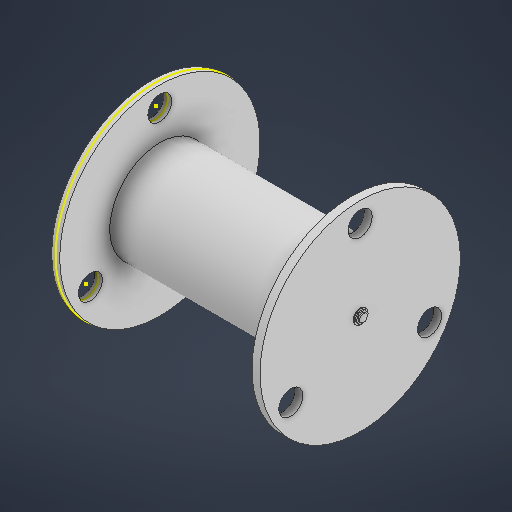
# Autodesk Inventor part: roller
Saved by Autodesk Inventor 2026.1 (Build 301233020, 233B)
## iProperties
Created: 2025-12-30
Part Number: roller
Material: Generic
Document SubType Name: Modeling
Designer: Austin Ngobeni
Density: 1 g/cm^3
Appearance: Default
Author: Austin Ngobeni
Autodesk Inventor part; units mm, degrees
ref_plane "YZ Plane" through (0, 0, 0) normal (1, 0, 0) x (0, 1, 0)
ref_plane "XZ Plane" through (0, 0, 0) normal (0, 1, 0) x (-1, 0, 0)
ref_plane "XY Plane" through (0, 0, 0) normal (0, 0, 1) x (1, 0, 0)
sketch "Sketch1" plane through (0, 0, 0) normal (1, 0, 0) x (0, 1, 0)
  circle A0 centre (0, 0) radius 125
  circle A1 centre (0, 0) radius 250
  circle A2 centre (0, 0) radius 15 construction
  line L0 (-12.825, -7.7795) -> (-13.1497, 7.217)
  line L1 (-13.1497, 7.217) -> (-0.3247, 14.9965)
  line L2 (-0.3247, 14.9965) -> (12.825, 7.7795)
  line L3 (12.825, 7.7795) -> (13.1497, -7.217)
  line L4 (13.1497, -7.217) -> (0.3247, -14.9965)
  line L5 (0.3247, -14.9965) -> (-12.825, -7.7795)
  circle A3 centre (0, 0) radius 17.5
  circle A4 centre (0, 0) radius 200 construction
  circle A5 centre (200, 0) radius 30
  circle A6 centre (-100, 173.2051) radius 30
  circle A7 centre (-100, -173.2051) radius 30
  circle A8 centre (0, 0) radius 10
  dimension "d2" = 30
  dimension "d12" = 400
  dimension "d0" = 250
  dimension "d1" = 500
  dimension "d3" = 35
  dimension "d13" = 60
  dimension "d16" = 360
  dimension "d20" = 20
  constraints: 12 end point, 7 centre point, 7 coincident, 1 horizontal alignment, 25 other
  measures "d0" diameter of A0
  measures "d1" diameter of A1
  measures "d3" diameter of A3
  measures "d13" diameter of A5
  measures "d20" diameter of A8
extrude "Extrusion1" add sketch "Sketch1" along normal mid plane 20 contours A0 | A1 | L0 L1 L2 L3 L4 L5 | A3 | A5 | A6 | A7 | A8
extrude "Extrusion2" add sketch "Sketch1" against normal blind 500 contours A0
extrude "Extrusion3" add sketch "Sketch1" along normal blind 15 contours L0 L1 L2 L3 L4 L5 | A8
extrude "Extrusion4" add sketch "Sketch1" along normal blind 12 contours A3
extrude "Extrusion5" cut sketch "Sketch1" along normal through all both and the other way through all contours A5 | A6 | A7
extrude "Extrusion6" add sketch "Sketch1" along normal blind 18 contours A8
sketch "Sketch2" plane through (-500, 0, 0) normal (-1, 0, 0) x (0, 0, 1)
  circle A0 centre (0, 0) radius 250 projected
  circle A1 centre (0, 200) radius 30 projected
  circle A2 centre (-173.2051, -100) radius 30 projected
  circle A3 centre (173.2051, -100) radius 30 projected
  circle A4 centre (0, 0) radius 17.5 projected
  circle A5 centre (0, 0) radius 10 projected
  line L0 (7.217, -13.1497) -> (-7.7795, -12.825) projected
  line L1 (-7.7795, -12.825) -> (-14.9965, 0.3247) projected
  line L2 (-14.9965, 0.3247) -> (-7.217, 13.1497) projected
  line L3 (-7.217, 13.1497) -> (7.7795, 12.825) projected
  line L4 (7.7795, 12.825) -> (14.9965, -0.3247) projected
  line L5 (14.9965, -0.3247) -> (7.217, -13.1497) projected
extrude "Extrusion7" add sketch "Sketch2" along normal mid plane 20 contours A0
extrude "Extrusion8" add sketch "Sketch2" along normal blind 18 contours A5
extrude "Extrusion9" cut sketch "Sketch2" along normal blind 17 contours A5 | L0 L1 L2 L3 L4 L5
extrude "Extrusion10" add sketch "Sketch2" along normal blind 12 contours A4 | A5 | L0 L1 L2 L3 L4 L5
extrude "Extrusion11" add sketch "Sketch2" along normal blind 15 contours A5 | L0 L1 L2 L3 L4 L5
body "Solid1"
